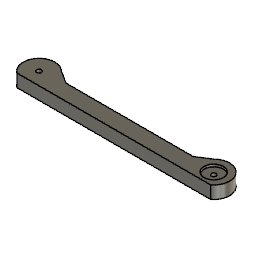
link_3 (Autodesk Fusion 360 design; units mm, degrees)
Autodesk Fusion 360 part; units mm, degrees
sketch "Sketch2" plane through (0, 0, 0) normal (0, 0, 1) x (1, 0, 0)
  line L0 (91, -8) -> (-31, -8)
  line L1 (-10, 2.005) -> (70, 2.005)
  line L2 (70, 2.005) -> (77.9321, 7.0743)
  line L3 (-10, 2.005) -> (-17.9321, 7.0743)
  arc A0 (-17.9321, 7.0743) -> (-31, -8) centre (-25, 0) ccw
  arc A1 (91, -8) -> (77.9321, 7.0743) centre (85, 0) ccw
  dimension "d20" = 20
  dimension "d21" = 20
  dimension "d22" = 110
  dimension "d24" = 10.005
  constraint horizontal L0
  constraint parallel L0 L1
  measures "d20" diameter of A0
  measures "d21" diameter of A1
  measures "d22" distance of A0.centre A1.centre
  measures "d24" distance of L0 L1
extrude "Extrude1" add sketch "Sketch2" along normal blind 8
sketch "Sketch3" plane through (0, 0, 8) normal (0, 0, 1) x (-1, 0, 0)
  line L0 (10, -2.005) -> (17.9321, -7.0743)
  arc A0 (17.9321, -7.0743) -> (31, 8) centre (25, 0) ccw
  line L1 (31, 8) -> (-91, 8)
  arc A1 (-91, 8) -> (-77.9321, -7.0743) centre (-85, 0) ccw
  line L2 (-77.9321, -7.0743) -> (-70, -2.005)
  line L3 (-70, -2.005) -> (10, -2.005)
  circle A2 centre (-85, 0) radius 6.1
  dimension "d28" = 12.2
  constraint concentric A1 A2
  measures "d28" diameter of A2
sketch "Sketch4" plane through (0, 0, 0) normal (0, 0, -1) x (1, 0, 0)
  line L0 (-17.9321, -7.0743) -> (-10, -2.005)
  line L1 (-10, -2.005) -> (70, -2.005)
  line L2 (70, -2.005) -> (77.9321, -7.0743)
  arc A0 (77.9321, -7.0743) -> (91, 8) centre (85, 0) ccw
  line L3 (91, 8) -> (-31, 8)
  arc A1 (-31, 8) -> (-17.9321, -7.0743) centre (-25, 0) ccw
  circle A2 centre (-25, 0) radius 6.1
  dimension "d32" = 12.2
  constraint concentric A1 A2
  measures "d32" diameter of A2
extrude "Extrude4" cut sketch "Sketch4" against normal blind 1.5 contours A2
extrude "Extrude5" cut sketch "Sketch3" against normal blind 1.5 contours A2
sketch "Sketch5" plane through (0, 0, 0) normal (0, 0, -1) x (1, 0, 0)
  circle A0 centre (-25, 0) radius 6.1
  line L0 (-17.9321, -7.0743) -> (-10, -2.005)
  line L1 (-10, -2.005) -> (70, -2.005)
  line L2 (70, -2.005) -> (77.9321, -7.0743)
  arc A1 (77.9321, -7.0743) -> (91, 8) centre (85, 0) ccw
  line L3 (91, 8) -> (-31, 8)
  arc A2 (-31, 8) -> (-17.9321, -7.0743) centre (-25, 0) ccw
  circle A3 centre (85, 0) radius 1.5
  dimension "d39" = 3
  constraint concentric A1 A3
  measures "d39" diameter of A3
extrude "Extrude7" cut sketch "Sketch5" against normal blind 13 contours A3
sketch "Sketch6" plane through (0, 0, 8) normal (0, 0, 1) x (-1, 0, 0)
  circle A0 centre (-85, 0) radius 6.1
  line L0 (10, -2.005) -> (17.9321, -7.0743)
  arc A1 (17.9321, -7.0743) -> (31, 8) centre (25, 0) ccw
  line L1 (31, 8) -> (-91, 8)
  arc A2 (-91, 8) -> (-77.9321, -7.0743) centre (-85, 0) ccw
  line L2 (-77.9321, -7.0743) -> (-70, -2.005)
  line L3 (-70, -2.005) -> (10, -2.005)
  circle A3 centre (25, 0) radius 1.5
  dimension "d44" = 3
  constraint concentric A1 A3
  measures "d44" diameter of A3
extrude "Extrude8" cut sketch "Sketch6" against normal blind 11 contours A3
component "arm1" placed x (1, 0, 0) y (0, 1, 0) z (0, 0, 1) at (0, 0, 0)
